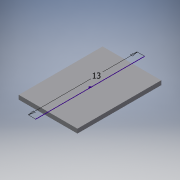
# Autodesk Inventor part: RubayetChip
Saved by Autodesk Inventor 2019 (Build 230136000, 136)
## iProperties
Created: 2019-06-10
Part Number: RubayetChip
Material: Generic
Document SubType Name: Modeling
Designer: aorfi
Density: 1 g/cm^3
Appearance: Default
Author: aorfi
Autodesk Inventor part; units mm, degrees
ref_plane "YZ Plane" through (0, 0, 0) normal (1, 0, 0) x (0, 1, 0)
ref_plane "XZ Plane" through (0, 0, 0) normal (0, 1, 0) x (-1, 0, 0)
ref_plane "XY Plane" through (0, 0, 0) normal (0, 0, 1) x (1, 0, 0)
sketch "Sketch1" plane through (0, 0, 0) normal (0, 1, 0) x (-1, 0, 0)
  line L0 (3.5, 5) -> (-3.5, 5)
  line L1 (-3.5, 5) -> (-3.5, -5)
  line L2 (-3.5, -5) -> (3.5, -5)
  line L3 (3.5, -5) -> (3.5, 5)
  line L4 (3.5, 5) -> (-3.5, -5) construction
  line L5 (-3.5, 5) -> (3.5, -5) construction
  point P0 (0, 0)
  dimension "d0" = 10
  dimension "d1" = 7
  constraints: 12 end point, 2 midpoint, 2 parallel, 1 horizontal, 1 perpendicular
  measures "d0" distance of L2.end L0.start
  measures "d1" distance of L1.end L2.end
extrude "Extrusion1" add sketch "Sketch1" along normal mid plane 0.5
sketch "Sketch2" plane through (0, 0.25, 0) normal (0, 1, 0) x (1, 0, 0)
  line L0 (0, -6.5) -> (0, 6.5)
  point P0 (0, 0)
  point P1 (0, 0)
  dimension "d4" = 13
  constraints: 2 end point, 1 coincident, 1 midpoint, 1 vertical
  measures "d4" distance of L0.start L0.end
body "Solid1"
